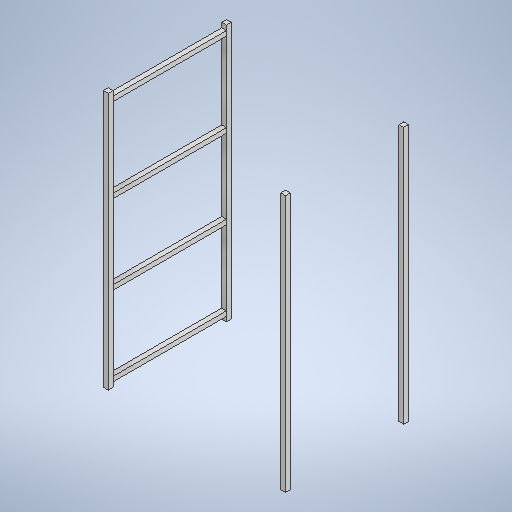
# Autodesk Inventor part: MM_00002.1.0
Saved by Autodesk Inventor 2025.3 (Build 293356000, 356)
## iProperties
Created: 2025-08-16
Part Number: MM_00002.1.0
Material: Generic
Document SubType Name: Modeling
Designer: FerreRo
Density: 1 g/cm^3
Appearance: Default
Author: FerreRo
Autodesk Inventor part; units mm, degrees
ref_plane "YZ Plane" through (0, 0, 0) normal (1, 0, 0) x (0, 1, 0)
ref_plane "XZ Plane" through (0, 0, 0) normal (0, 1, 0) x (-1, 0, 0)
ref_plane "XY Plane" through (0, 0, 0) normal (0, 0, 1) x (1, 0, 0)
sketch "Sketch1" plane through (0, 0, 0) normal (0, 0, 1) x (1, 0, 0)
  line L0 (-300, 0) -> (300, 0)
  line L1 (300, 0) -> (300, 835)
  line L2 (300, 835) -> (-300, 835)
  line L3 (-300, 835) -> (-300, 0)
  point P0 (0, 0)
  point P1 (0, 0)
  dimension "d0" = 835
  dimension "d1" = 600
  constraints: 8 end point, 2 parallel, 1 coincident, 1 horizontal, 1 midpoint, 1 perpendicular
  measures "d0" distance of L0.end L1.end
  measures "d1" distance of L0.start L0.end
sketch "Sketch2" plane through (0, 0, 0) normal (0, 1, 0) x (-1, 0, 0)
  line L0 (300, -200) -> (-300, -200)
  line L1 (-300, -200) -> (-300, 200)
  line L2 (-300, 200) -> (300, 200)
  line L3 (300, 200) -> (300, -200)
  line L4 (300, -200) -> (-300, 200) construction
  line L5 (-300, -200) -> (300, 200) construction
  point P0 (0, 0)
  dimension "d2" = 600
  dimension "d3" = 400
  constraints: 12 end point, 2 midpoint, 2 parallel, 1 horizontal, 1 perpendicular
  measures "d2" distance of L0.start L0.end
  measures "d3" distance of L2.end L0.start
sketch "Sketch4" plane through (0, 0, 0) normal (0, 1, 0) x (-1, 0, 0)
  line L0 (-300, 200) -> (300, 200) projected
  line L1 (300, 200) -> (300, -200) projected
  line L2 (300, -200) -> (-300, -200) projected
  line L3 (-300, -200) -> (-300, 200) projected
  point P0 (0, 0)
extrude "Extrusion2" add sketch "Sketch4" along normal blind 15
sketch "Sketch5" plane through (0, 15, 0) normal (0, 1, 0) x (1, 0, 0)
  line L0 (-285, 200) -> (-270, 200)
  line L1 (-270, 200) -> (-270, 185)
  line L2 (-270, 185) -> (-285, 185)
  line L3 (-285, 185) -> (-285, 200)
  line L4 (-300, 200) -> (-300, -200) construction
  line L5 (300, 200) -> (-300, 200) construction
  line L6 (-270, -185) -> (-285, -185)
  line L7 (-270, -170) -> (-270, -185)
  line L8 (-285, -170) -> (-270, -170)
  line L9 (-285, -185) -> (-285, -170)
  line L10 (285, 185) -> (270, 185)
  line L11 (285, 200) -> (285, 185)
  line L12 (270, 200) -> (285, 200)
  line L13 (270, 185) -> (270, 200)
  line L14 (285, -185) -> (270, -185)
  line L15 (285, -170) -> (285, -185)
  line L16 (270, -170) -> (285, -170)
  line L17 (270, -185) -> (270, -170)
  point P0 (0, 0)
  dimension "d31" = 15
  dimension "d32" = 15
  dimension "d33" = 0
  dimension "d34" = 15
  dimension "d37" = 370
  dimension "d40" = 555
  constraints: 32 end point, 2 horizontal, 2 parallel, 1 perpendicular, 1 vertical, 24 other
  measures "d31" distance of L0.end L1.end
  measures "d32" distance of L0.start L0.end
  measures "d33" distance between parallel lines of L5 L0
  measures "d34" distance between parallel lines of L4 L3
  measures "d37" distance of L1.end L6.start
  measures "d40" distance of L1.end L10.start
pattern_linear "Rectangular Pattern1" count 2 spacing 820 along (0, 1, 0)
extrude "Extrusion3" add sketch "Sketch5" along normal up to surface (805 mm away) separate body
sketch "Sketch6" plane through (-285, 15, -185) normal (0, 0, 1) x (1, 0, 0)
  line L0 (0, 278.3333) -> (15, 278.3333)
  line L1 (15, 278.3333) -> (15, 263.3333)
  line L2 (15, 263.3333) -> (0, 263.3333)
  line L3 (0, 263.3333) -> (0, 278.3333)
  line L4 (15, 0) -> (15, 805) construction
  line L5 (0, 0) -> (0, 805) construction
  line L6 (0, 526.6667) -> (15, 526.6667)
  line L7 (15, 526.6667) -> (15, 511.6667)
  line L8 (15, 511.6667) -> (0, 511.6667)
  line L9 (0, 511.6667) -> (0, 526.6667)
  line L10 (0, 30) -> (15, 30)
  line L11 (15, 30) -> (15, 15)
  line L12 (15, 15) -> (0, 15)
  line L13 (0, 15) -> (0, 30)
  line L14 (0, 0) -> (15, 0) construction
  line L15 (0, 790) -> (15, 790)
  line L16 (15, 790) -> (15, 775)
  line L17 (15, 775) -> (0, 775)
  line L18 (0, 775) -> (0, 790)
  line L19 (15, 805) -> (0, 805) construction
  point P0 (285, -15)
  dimension "d46" = 15
  dimension "d47" = 15
  dimension "d49" = 15
  dimension "d52" = 248.3333
  dimension "d53" = 248.3333
  dimension "d54" = 15
  dimension "d65" = 15
  dimension "d66" = 15
  dimension "d67" = 248.3333
  dimension "d68" = 15
  constraints: 32 end point, 8 parallel, 7 collinear, 4 horizontal, 4 perpendicular
  measures "d46" distance of L0.start L0.end
  measures "d47" distance between parallel lines of L0 L2
  measures "d49" distance between parallel lines of L8 L6
  measures "d52" distance between parallel lines of L2 L12
  measures "d53" distance between parallel lines of L8 L2
  measures "d54" distance of L15.end L16.end
  measures "d65" distance between parallel lines of L10 L12
  measures "d66" distance between parallel lines of L14 L12
  measures "d67" distance between parallel lines of L17 L6
  measures "d68" distance between parallel lines of L19 L15
extrude "Extrusion4" add sketch "Sketch6" along normal up to surface (355 mm away) separate body
mirror "Mirror1" about plane through (0, 0, 0) normal (1, 0, 0) bodies 3 separate body
sketch "Sketch7" plane through (-270, 15, 185) normal (1, 0, 0) x (0, 0, -1)
  line L0 (0, 805) -> (15, 805)
  line L1 (15, 805) -> (15, 790)
  line L2 (15, 790) -> (0, 790)
  line L3 (0, 790) -> (0, 805)
  line L4 (0, 0) -> (0, 805) construction
  line L5 (15, 805) -> (0, 805) projected
  line L6 (0, 15) -> (15, 15)
  line L7 (15, 15) -> (15, 0)
  line L8 (15, 0) -> (0, 0)
  line L9 (0, 0) -> (0, 15)
  line L10 (0, 0) -> (0, 805) construction
  line L11 (0, 0) -> (15, 0) construction
  line L12 (385, 805) -> (370, 805)
  line L13 (370, 805) -> (370, 790)
  line L14 (370, 790) -> (385, 790)
  line L15 (385, 790) -> (385, 805)
  line L16 (385, 0) -> (385, 805) construction
  line L17 (385, 805) -> (370, 805) projected
  line L18 (385, 15) -> (370, 15)
  line L19 (370, 15) -> (370, 0)
  line L20 (370, 0) -> (385, 0)
  line L21 (385, 0) -> (385, 15)
  line L22 (370, 0) -> (385, 0) projected
  point P0 (185, -15)
  dimension "d57" = 15
  dimension "d58" = 15
  dimension "d59" = 0
  dimension "d60" = 15
  dimension "d61" = 15
  dimension "d62" = 0
  dimension "d69" = 15
  dimension "d70" = 15
  dimension "d71" = 15
  dimension "d72" = 15
  constraints: 32 end point, 8 parallel, 6 collinear, 4 horizontal, 4 perpendicular
  measures "d57" distance of L0.start L0.end
  measures "d58" distance of L2.end L0.start
  measures "d59" distance between parallel lines of L5 L0
  measures "d60" distance of L8.end L6.start
  measures "d61" distance of L6.start L6.end
  measures "d62" distance between parallel lines of L11 L8
  measures "d69" distance of L12.start L12.end
  measures "d70" distance of L14.end L12.start
  measures "d71" distance of L20.end L18.start
  measures "d72" distance of L18.start L18.end
extrude "Extrusion5" add sketch "Sketch7" along normal up to surface (540 mm away) separate body
sketch "Sketch8" plane through (285, 15, -185) normal (1, 0, 0) x (0, 0, -1)
  line L0 (-385, 0) -> (15, 0)
  line L1 (15, 0) -> (15, 805)
  line L2 (15, 805) -> (-385, 805)
  line L3 (-385, 805) -> (-385, 0)
  point P0 (-185, -15)
  point P1 (-385, 805)
  point P2 (15, 0)
  constraints: 8 end point, 2 parallel, 1 horizontal, 1 perpendicular
extrude "Extrusion6" add sketch "Sketch8" along normal blind 15 separate body
mirror "Mirror2" about plane through (0, 0, 0) normal (1, 0, 0) bodies 6 separate body
sketch "Sketch9" plane through (-300, 0, 200) normal (0, 0, 1) x (1, 0, 0)
  line L0 (15, 820) -> (585, 820)
  line L1 (585, 820) -> (585, 15)
  line L2 (585, 15) -> (15, 15)
  line L3 (15, 15) -> (15, 820)
  point P0 (300, 0)
  point P1 (15, 15)
  constraints: 8 end point, 2 parallel, 1 horizontal, 1 perpendicular
extrude "Extrusion7" add sketch "Sketch9" against normal blind 15 separate body
sketch "Sketch10" plane through (300, 820, -200) normal (0, 0, -1) x (-1, 0, 0)
  line L0 (0, 15) -> (600, 15)
  line L1 (600, 15) -> (600, -820)
  line L2 (600, -820) -> (0, -820)
  line L3 (0, -820) -> (0, 15)
  point P0 (300, -820)
  point P1 (0, -820)
  constraints: 8 end point, 2 parallel, 1 horizontal, 1 perpendicular
extrude "Extrusion8" add sketch "Sketch10" along normal blind 15 separate body
move or copy body "Move Body1" bodies to move or copy 9 copy no translate (-300, 0, -5)
sketch "Sketch11" plane through (270, 293.3333, -185) normal (0, 1, 0) x (1, 0, 0)
  line L0 (15, -355) -> (-555, -355)
  line L1 (-555, -355) -> (-555, 0)
  line L2 (-555, 0) -> (15, 0)
  line L3 (15, 0) -> (15, -355)
  point P0 (-270, -185)
  constraints: 8 end point, 2 parallel, 1 horizontal, 1 perpendicular
extrude "Extrusion9" add sketch "Sketch11" along normal blind 15 separate body
sketch "Sketch12" plane through (270, 541.6667, -185) normal (0, 1, 0) x (1, 0, 0)
  line L0 (15, -355) -> (-555, -355)
  line L1 (-555, -355) -> (-555, 0)
  line L2 (-555, 0) -> (15, 0)
  line L3 (15, 0) -> (15, -355)
  point P0 (-270, -185)
  constraints: 8 end point, 2 parallel, 1 horizontal, 1 perpendicular
extrude "Extrusion10" add sketch "Sketch12" along normal blind 15 separate body
sketch "Sketch13" plane through (0, 0, 0) normal (0, -1, 0) x (1, 0, 0)
  line L0 (250, -200) -> (235, -200)
  line L1 (235, -200) -> (235, 200)
  line L2 (235, 200) -> (250, 200)
  line L3 (250, 200) -> (250, -200)
  line L4 (300, -200) -> (-300, -200) projected
  line L5 (-300, 200) -> (300, 200) projected
  line L6 (300, 200) -> (300, -200) projected
  line L7 (-235, 200) -> (-250, 200)
  line L8 (-250, 200) -> (-250, -200)
  line L9 (-250, -200) -> (-235, -200)
  line L10 (-235, -200) -> (-235, 200)
  line L11 (-300, -200) -> (-300, 200) projected
  point P0 (0, 0)
  point P1 (-235, -200)
  point P2 (-250, -200)
  dimension "d86" = 15
  dimension "d87" = 50
  dimension "d88" = 15
  dimension "d89" = 50
  constraints: 16 end point, 4 collinear, 4 parallel, 2 horizontal, 2 perpendicular
  measures "d86" distance of L0.start L0.end
  measures "d87" distance between parallel lines of L6 L3
  measures "d88" distance between parallel lines of L8 L10
  measures "d89" distance between parallel lines of L8 L11
extrude "Extrusion11" add sketch "Sketch13" along normal blind 15 separate body contours L0 L1 L2 L3 | L4 L8 L5 L10
equation "\"d2\" = d1"
equation "\"d53\" = d52"
equation "\"d67\" = d53"
body "Solid1"
